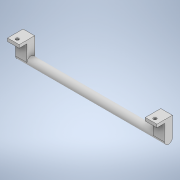
# Autodesk Inventor part: Supporting-Rod
Saved by Autodesk Inventor 2021 (Build 250183000, 183)
## iProperties
Created: 2021-02-22
Part Number: Supporting-Rod
Material: Generic
Document SubType Name: Modeling
Designer: chris
Density: 1 g/cm^3
Appearance: Default
Author: chris
Autodesk Inventor part; units mm, degrees
ref_plane "YZ Plane" through (0, 0, 0) normal (1, 0, 0) x (0, 1, 0)
ref_plane "XZ Plane" through (0, 0, 0) normal (0, 1, 0) x (-1, 0, 0)
ref_plane "XY Plane" through (0, 0, 0) normal (0, 0, 1) x (1, 0, 0)
sketch "Sketch1" plane through (0, 0, 0) normal (0, 0, 1) x (1, 0, 0)
  point P0 (0, 0)
sketch "Sketch2" plane through (0, 0, 0) normal (1, 0, 0) x (0, 1, 0)
  circle A0 centre (0, 0) radius 5
  dimension "d0" = 10
  constraints: 1 centre point, 1 coincident
  measures "d0" diameter of A0
extrude "Extrusion1" add sketch "Sketch2" along normal blind 96.4
sketch "Sketch3" plane through (0, 0, 0) normal (-1, 0, 0) x (0, 0, 1)
  circle A0 centre (0, 0) radius 5 projected
  line L0 (-5, 0) -> (5, 0)
  arc A1 (5, 0) -> (-5, 0) centre (0, 0) ccw
  dimension "d3" = 5
  constraints: 4 point on circle, 2 end point, 1 centre point, 1 concentric, 1 horizontal
  measures "d3" distance edge to line of A0 L0
extrude "Extrusion2" cut sketch "Sketch3" against normal blind 15 contours L0 A0 picked at (1.2475, 1.1052)
sketch "Sketch4" plane through (0, 0, 5) normal (0, 1, 0) x (1, 0, 0)
  line L0 (15, 0) -> (0, 0) projected
  line L1 (15, 0) -> (15, 10) projected
  line L2 (0, 0) -> (15, 0)
  line L3 (15, 0) -> (15, 10)
  line L4 (15, 10) -> (0, 10)
  line L5 (0, 10) -> (0, 0)
  point P0 (0, 5)
  constraints: 8 end point, 2 parallel, 1 horizontal, 1 perpendicular
extrude "Extrusion3" add sketch "Sketch4" along normal blind 25
sketch "Sketch5" plane through (0, 0, 5) normal (0, 0, 1) x (1, 0, 0)
  line L0 (0, 0) -> (0, 25) projected
  line L1 (0, 25) -> (15, 25)
  line L2 (15, 25) -> (15, 21)
  line L3 (15, 21) -> (0, 21)
  line L4 (0, 21) -> (0, 25)
  point P0 (0, 21)
  dimension "d8" = 4
  dimension "d9" = 15
  constraints: 8 end point, 2 parallel, 1 horizontal, 1 perpendicular
  measures "d8" distance of L1.end L2.end
  measures "d9" distance of L2.end L3.end
extrude "Extrusion4" add sketch "Sketch5" along normal blind 10
sketch "Sketch6" plane through (0, 21, 5) normal (0, -1, 0) x (1, 0, 0)
  circle A0 centre (7.5, 5) radius 3.5
  line L0 (0, 0) -> (0, 10) projected
  line L1 (15, 0) -> (0, 0) projected
  point P0 (0, -5)
  dimension "d12" = 7
  dimension "d13" = 7.5
  dimension "d14" = 5
  constraints: 1 centre point
  measures "d12" diameter of A0
  measures "d13" distance from line of L0 A0.centre
  measures "d14" distance from line of L1 A0.centre
extrude "Extrusion5" cut sketch "Sketch6" against normal blind 2.8
sketch "Sketch7" plane through (7.5, 23.8, 10) normal (0, -1, 0) x (1, 0, 0)
  circle A0 centre (0, 0) radius 2
  line L0 (-7.5, -5) -> (-7.5, 5) projected
  line L1 (7.5, -5) -> (-7.5, -5) projected
  point P0 (-7.5, -10)
  dimension "d17" = 7.5
  dimension "d18" = 5
  dimension "d19" = 4
  constraints: 1 centre point
  measures "d17" distance from line of L0 A0.centre
  measures "d18" distance from line of L1 A0.centre
  measures "d19" diameter of A0
extrude "Extrusion6" cut sketch "Sketch7" against normal through all
mirror "Mirror1" about plane through (96.4, 0, 0) normal (1, 0, 0) of "Extrusion5", "Extrusion6", "Extrusion4", "Extrusion3", "Extrusion1"
body "Solid1"
